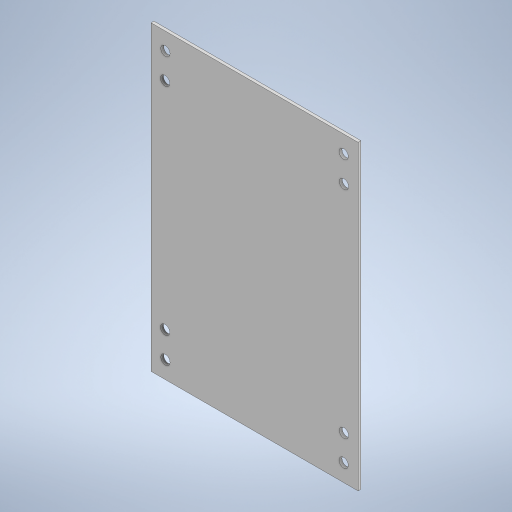
# Autodesk Inventor part: side1
Saved by Autodesk Inventor 2023 (Build 270158000, 158)
## iProperties
Created: 2023-05-28
Part Number: side1
Material: 一般
Document SubType Name: Sheet Metal
Designer: 310611102
Density: 1 g/cm^3
Sheet Metal Rule: Default_mm
Appearance: 預設
Author: 310611102
Autodesk Inventor part; units mm, degrees
ref_plane "YZ Plane" through (0, 0, 0) normal (1, 0, 0) x (0, 1, 0)
ref_plane "XZ Plane" through (0, 0, 0) normal (0, 1, 0) x (-1, 0, 0)
ref_plane "XY Plane" through (0, 0, 0) normal (0, 0, 1) x (1, 0, 0)
sketch "Sketch1" plane through (0, 0, 0) normal (0, 0, 1) x (1, 0, 0)
  line L0 (-36, 52.5) -> (36, 52.5)
  line L1 (36, 52.5) -> (36, -52.5)
  line L2 (36, -52.5) -> (-36, -52.5)
  line L3 (-36, -52.5) -> (-36, 52.5)
  line L4 (-36, 52.5) -> (36, -52.5) construction
  line L5 (36, 52.5) -> (-36, -52.5) construction
  circle A0 centre (31.1, -37.5) radius 1.6
  line L6 (0, 0) -> (12.8976, 0)
  line L7 (0, 0) -> (0, 11.3109)
  circle A1 centre (-31.1, -37.5) radius 1.6
  circle A2 centre (31.1, 37.5) radius 1.6
  circle A3 centre (-31.1, 37.5) radius 1.6
  circle A4 centre (-31, -46.5) radius 1.6
  circle A5 centre (-31, 46.5) radius 1.6
  circle A6 centre (31, -46.5) radius 1.6
  circle A7 centre (31, 46.5) radius 1.6
  dimension "d0" = 72
  dimension "d1" = 105
  dimension "d2" = 3.2
  dimension "d3" = 4.9
  dimension "d4" = 15
  dimension "d6" = 3.2
  dimension "d7" = 6
  dimension "d8" = 5
  measures "d0" distance of L1.end L2.end
  measures "d1" distance of L0.end L1.end
  measures "d2" diameter of A0
  measures "d3" distance from line of L1 A0.centre
  measures "d4" distance from line of L2 A0.centre
  measures "d6" diameter of A4
  measures "d7" distance from line of L2 A4.centre
  measures "d8" distance from line of L3 A4.centre
extrude "Plate1" add sketch "Sketch1" along normal blind 1
equation "\"d5\" = 厚度"
equation "\"折彎半徑\" = 厚度"
equation "\"折彎離隙寬度\" = 厚度"
equation "\"折彎離隙深度\" = 0.5 * 厚度"
equation "\"轉角離隙大小\" = 4 * 厚度"
equation "\"最小剩餘\" = 2 * 厚度"
equation "\"轉移半徑\" = 折彎半徑"
equation "\"Jacobi半徑大小\" = 折彎半徑"
equation "\"間隙大小\" = 厚度"
equation "\"厚度\" = 1"
body "Solid1"
